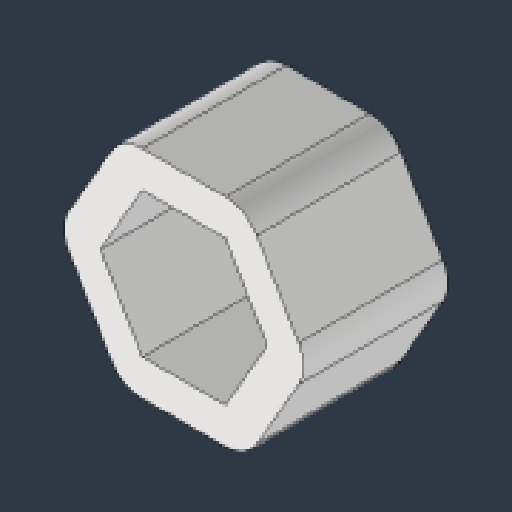
# Autodesk Inventor part: 1-2in_spacer
Saved by Autodesk Inventor 2024.3 (Build 283343000, 343)
## iProperties
Created: 2025-03-10
Part Number: 1-2in_spacer
Material: Generic
Document SubType Name: Modeling
Designer: Marcus Tannini
Density: 1 g/cm^3
Appearance: Default
Author: Marcus Tannini
Autodesk Inventor part; units mm, degrees
ref_plane "YZ Plane" through (0, 0, 0) normal (1, 0, 0) x (0, 1, 0)
ref_plane "XZ Plane" through (0, 0, 0) normal (0, 1, 0) x (-1, 0, 0)
ref_plane "XY Plane" through (0, 0, 0) normal (0, 0, 1) x (1, 0, 0)
sketch "Sketch1" plane through (0, 0, 0) normal (0, 0, 1) x (1, 0, 0)
  line L0 (-3.6735, 6.3627) -> (3.6735, 6.3627)
  line L1 (3.6735, 6.3627) -> (7.347, 0)
  line L2 (7.347, 0) -> (3.6735, -6.3627)
  line L3 (3.6735, -6.3627) -> (-3.6735, -6.3627)
  line L4 (-3.6735, -6.3627) -> (-7.347, 0)
  line L5 (-7.347, 0) -> (-3.6735, 6.3627)
  line L6 (-15.4185, 0) -> (15.4185, 0) construction
  line L7 (-5.5066, 9.5377) -> (5.5066, 9.5377)
  line L8 (5.5066, 9.5377) -> (11.0132, 0)
  line L9 (11.0132, 0) -> (5.5066, -9.5377)
  line L10 (5.5066, -9.5377) -> (-5.5066, -9.5377)
  line L11 (-5.5066, -9.5377) -> (-11.0132, 0)
  line L12 (-11.0132, 0) -> (-5.5066, 9.5377)
  point P0 (0, 0)
  point P1 (0, 0)
  point P2 (0, 0)
  dimension "d0" = 12.7254
  dimension "d1" = 3.175
  constraints: 24 end point, 2 coincident, 2 parallel, 26 other
  measures "d0" distance between parallel lines of L3 L0
  measures "d1" distance between parallel lines of L0 L7
extrude "Extrusion1" add sketch "Sketch1" along normal blind 12.7
fillet "Fillet1" radius 3.175 6 edges at (5.5066, -9.5377, 6.35) (-5.5066, -9.5377, 6.35) (11.0132, 0, 6.35) (-11.0132, 0, 6.35) (-5.5066, 9.5377, 6.35) (5.5066, 9.5377, 6.35)
body "Solid1"
